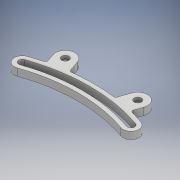
# Autodesk Inventor part: reverse gear gear link
Saved by Autodesk Inventor 2017 (Build 210142000, 142)
## iProperties
Created: 2018-11-06
Part Number: reverse gear gear link
Material: Generic
Document SubType Name: Modeling
Designer: User
Density: 1 g/cm^3
Appearance: Default
Author: User
Autodesk Inventor part; units mm, degrees
ref_plane "YZ Plane" through (0, 0, 0) normal (1, 0, 0) x (0, 1, 0)
ref_plane "XZ Plane" through (0, 0, 0) normal (0, 1, 0) x (-1, 0, 0)
ref_plane "XY Plane" through (0, 0, 0) normal (0, 0, 1) x (1, 0, 0)
sketch "Sketch3" plane through (0, 0, 0) normal (0, 0, 1) x (1, 0, 0)
  line L0 (18.7781, 73.7011) -> (17.3583, 69.6186)
  line L1 (22.5, 64.6993) -> (23.5675, 67.769) construction
  line L2 (11.2219, 76.3289) -> (9.4139, 71.1298)
  arc A0 (22.0073, 63.2825) -> (22.9927, 66.1161) centre (22.5, 64.6993) ccw
  circle A1 centre (22.5, 64.6993) radius 1.5 construction
  arc A2 (21.4325, 61.6296) -> (23.5675, 67.769) centre (22.5, 64.6993) ccw
  arc A3 (21.4325, 61.6296) -> (-21.4325, 61.6296) centre (0, 0) ccw
  arc A4 (22.0073, 63.2825) -> (-22.0073, 63.2825) centre (0, 0) ccw
  arc A5 (22.5, 64.6993) -> (-22.5, 64.6993) centre (0, 0) ccw construction
  arc A6 (23.5675, 67.769) -> (-23.5675, 67.769) centre (0, 0) ccw
  circle A7 centre (0, 0) radius 76.5 construction
  circle A8 centre (0, 0) radius 68.5 construction
  arc A9 (22.9927, 66.1161) -> (-22.9927, 66.1161) centre (0, 0) ccw
  circle A10 centre (-22.5, 64.6993) radius 1.5 construction
  arc A11 (-22.9927, 66.1161) -> (-22.0073, 63.2825) centre (-22.5, 64.6993) ccw
  arc A12 (-23.5675, 67.769) -> (-21.4325, 61.6296) centre (-22.5, 64.6993) ccw
  arc A13 (18.7781, 73.7011) -> (11.2219, 76.3289) centre (15, 75.015) ccw
  dimension "d32" = 153
  dimension "d33" = 8
  dimension "d34" = 3.25
  dimension "d35" = 45
  dimension "d36" = 22.5
  dimension "d37" = 3
  dimension "d38" = 8
  dimension "d39" = 15
  dimension "d40" = 0
  dimension "d41" = 71.75
  constraints: 24 point on circle, 13 centre point, 8 tangent, 6 end point, 4 coincident, 2 equal radius, 2 parallel, 6 other
  measures "d34" radius of A2
  measures "d35" distance of A5.end A0.centre
  measures "d36" horizontal distance of point (0, 0) A0.centre
  measures "d37" diameter of A1
  measures "d38" diameter of A13
  measures "d39" horizontal distance of A3.centre A13.centre
  measures "d40" distance from line of point (0, 0) L1
  measures "d41" distance of point (0, 0) L1.end
extrude "Extrusion4" add sketch "Sketch3" along normal mid plane 3 contours A6 A2 A3 A12
extrude "Extrusion5" add sketch "Sketch3" along normal mid plane 3 contours L0 A6 L2 A13
sketch "Sketch5" plane through (0, 0, -1.5) normal (0, 0, -1) x (-1, 0, 0)
  circle A0 centre (-15, 75.015) radius 1.5
  arc A1 (-11.2219, 76.3289) -> (-18.7781, 73.7011) centre (-15, 75.015) ccw
  line L0 (-18.7781, 73.7011) -> (-17.3583, 69.6186)
  point P0 (0, 0)
  point P1 (0, 0)
  dimension "d46" = 3
  dimension "d47" = 0
  dimension "d48" = 4
  constraints: 2 centre point, 2 end point, 2 point on circle
  measures "d46" diameter of A0
  measures "d47" distance of A1.centre A0.centre
  measures "d48" distance from line of L0 A0.centre
hole "Hole1" at (15, 75.015, -1.5) direction (0, 0, 1) diameter 3 end through all countersink diameter 6.5 countersink angle 90
mirror "Mirror1" about plane through (0, 0, 0) normal (1, 0, 0) of "Hole1", "Extrusion5"
fillet "Fillet1" radius 1 4 edges at (-17.3583, 69.6186, 0) (-9.4139, 71.1298, 0) (17.3583, 69.6186, 0) (9.4139, 71.1298, 0)
body "Solid3"
